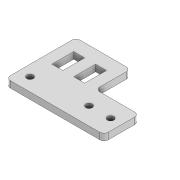
# Autodesk Inventor part: Bar_connection_plate
Saved by Autodesk Inventor 2022 (Build 260153000, 153)
## iProperties
Created: 2022-08-24
Part Number: Bar_connection_plate
Material: Generic
Document SubType Name: Modeling
Designer: dell
Density: 1 g/cm^3
Appearance: Default
Author: dell
Autodesk Inventor part; units mm, degrees
ref_plane "YZ Plane" through (0, 0, 0) normal (1, 0, 0) x (0, 1, 0)
ref_plane "XZ Plane" through (0, 0, 0) normal (0, 1, 0) x (-1, 0, 0)
ref_plane "XY Plane" through (0, 0, 0) normal (0, 0, 1) x (1, 0, 0)
sketch "Sketch1" plane through (0, 0, 0) normal (0, 1, 0) x (-1, 0, 0)
  circle A0 centre (0, 0) radius 1.5
  circle A1 centre (25, 2) radius 1.5
  line L0 (30, 8) -> (-14.9, 8)
  line L1 (-14.9, 8) -> (-14.9, -24)
  line L2 (-14.9, -24) -> (30, -24)
  line L3 (30, -24) -> (30, 8)
  line L4 (-14.9, -8) -> (30, -8) construction
  circle A2 centre (-9.9, 0) radius 1.5
  line L5 (25, -8) -> (20, -8)
  line L6 (20, -8) -> (20, -18)
  line L7 (20, -18) -> (25, -18)
  line L8 (25, -18) -> (25, -8)
  line L9 (20, -8) -> (20, -18)
  line L10 (20, -18) -> (15, -18)
  line L11 (15, -18) -> (15, -8)
  line L12 (15, -8) -> (20, -8)
  line L13 (15, -8) -> (15, -18)
  line L14 (15, -18) -> (10, -18)
  line L15 (10, -18) -> (10, -8)
  line L16 (10, -8) -> (15, -8)
  line L17 (5, -24) -> (-14.9, -24)
  line L18 (-14.9, -24) -> (-14.9, -8)
  line L19 (-14.9, -8) -> (5, -8)
  line L20 (5, -8) -> (5, -24)
  dimension "d0" = 3
  dimension "d1" = 3
  dimension "d3" = 25
  dimension "d4" = 2
  dimension "d5" = 8
  dimension "d6" = 6
  dimension "d7" = 5
  dimension "d9" = 3
  dimension "d10" = 9.9
  dimension "d11" = 5
  dimension "d12" = 10
  dimension "d13" = 5
  dimension "d14" = 5
  dimension "d15" = 5
  dimension "d16" = 6
  dimension "d19" = 5
  constraints: 42 end point, 12 equal length, 6 perpendicular, 3 centre point, 3 horizontal, 3 point on line, 2 midpoint, 1 coincident, 1 horizontal alignment
  measures "d0" diameter of A0
  measures "d1" diameter of A1
  measures "d3" horizontal distance of point (0, 0) A1.centre
  measures "d4" vertical distance of point (0, 0) A1.centre
  measures "d5" distance from line of point (0, 0) L4
  measures "d6" distance from line of L0 A1.centre
  measures "d7" distance from line of A1.centre L3
  measures "d9" diameter of A2
  measures "d10" distance of point (0, 0) A2.centre
  measures "d11" distance from line of L1 A2.centre
  measures "d12" distance of L5.end L6.end
  measures "d13" distance of L6.end L7.end
  measures "d14" distance of L6.end L10.end
  measures "d15" distance of L10.end L14.end
  measures "d16" distance between parallel lines of L7 L2
  measures "d19" horizontal distance of L14.end L17.start
extrude "Extrusion1" add sketch "Sketch1" along normal blind 3 contours L3 L2 L20 L19 L1 L0 | L6 L10 L11 L12
fillet "Fillet1" radius 2 6 edges at (-30, 1.5, 8) (-30, 1.5, -24) (-5, 1.5, -24) (14.9, 1.5, -8) (14.9, 1.5, 8) (-5, 1.5, -8)
body "Solid1"
